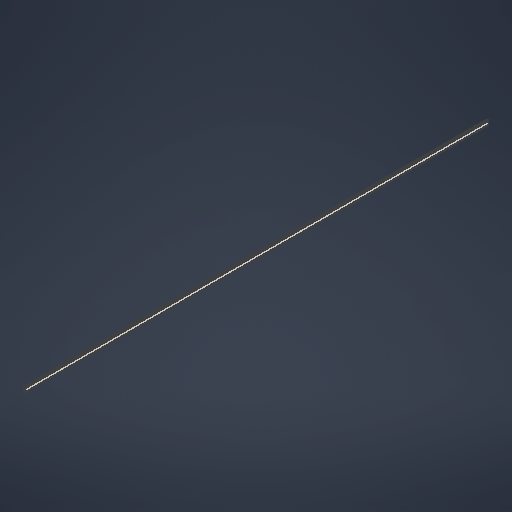
# Autodesk Inventor part: SP40-04A TRAVESAÑO CENTRAL
Saved by Autodesk Inventor 2025 (Build 290162000, 162)
## iProperties
Created: 2026-01-20
Part Number: SP40-04A TRAVESAÑO CENTRAL
Material: Aluminio
Document SubType Name: Modeling
Designer: ROLANDO
Density: 2.7 g/cm^3
Appearance: Satinado
Author: ROLANDO
Autodesk Inventor part; units mm, degrees
ref_plane "YZ Plane" through (0, 0, 0) normal (1, 0, 0) x (0, 1, 0)
ref_plane "XZ Plane" through (0, 0, 0) normal (0, 1, 0) x (-1, 0, 0)
ref_plane "XY Plane" through (0, 0, 0) normal (0, 0, 1) x (1, 0, 0)
sketch "Boceto1" plane through (0, 0, 0) normal (0, 0, 1) x (1, 0, 0)
  line L0 (-4.7609, 13.4664) -> (-4.7609, -16.5336)
  line L1 (-4.7609, -16.5336) -> (0.4391, -16.5336)
  line L2 (0.4391, -16.5336) -> (0.4391, -14.8936)
  line L3 (-0.9609, -15.1336) -> (-3.3609, -15.1336)
  line L4 (-3.3609, -15.1336) -> (-3.3609, -3.0336)
  line L5 (-2.8609, -2.5336) -> (17.5391, -2.5336)
  line L6 (18.0391, -3.0336) -> (18.0391, -7.2336)
  line L7 (18.0391, -7.2336) -> (14.2391, -7.2336)
  line L8 (14.2391, -7.2336) -> (14.2391, -8.8736)
  line L9 (14.9333, -9.8836) -> (15.6391, -9.8836)
  line L10 (15.6391, -9.8836) -> (15.6391, -8.6336)
  line L11 (15.6391, -8.6336) -> (18.0391, -8.6336)
  line L12 (18.0391, -8.6336) -> (18.0391, -15.1336)
  line L13 (18.0391, -15.1336) -> (15.6391, -15.1336)
  line L14 (15.6391, -15.1336) -> (15.6391, -13.8836)
  line L15 (15.6391, -13.8836) -> (14.9333, -13.8836)
  line L16 (14.2391, -14.8936) -> (14.2391, -16.5336)
  line L17 (14.2391, -16.5336) -> (19.4391, -16.5336)
  line L18 (19.4391, -16.5336) -> (19.4391, 13.4664)
  line L19 (-3.3609, 13.4664) -> (-3.3609, -0.6336)
  line L20 (18.0391, -0.6336) -> (18.0391, 13.4664)
  line L21 (7.3391, 11.7517) -> (7.3391, -2.5336) construction
  arc A0 (6.2391, 3.4216) -> (8.4391, 3.4216) centre (7.3391, 1.5164) ccw
  line L22 (-8.4881, 13.4664) -> (24.4446, 13.4664) construction
  line L23 (4.9522, 1.2664) -> (5.1534, 1.2664)
  line L24 (4.9522, 1.7664) -> (5.1534, 1.7664)
  line L25 (-2.8609, -1.1336) -> (3.8304, -1.1336)
  line L26 (10.8478, -1.1336) -> (17.5391, -1.1336)
  line L27 (4.0797, 1.5164) -> (9.7739, 1.5164) construction
  line L28 (9.726, 1.2664) -> (9.5249, 1.2664)
  line L29 (9.726, 1.7664) -> (9.5249, 1.7664)
  line L30 (7.5891, -0.8706) -> (7.5891, -0.6694)
  line L31 (7.0891, -0.8706) -> (7.0891, -0.6694)
  arc A1 (7.0891, -0.8706) -> (7.5891, -0.8706) centre (7.3391, 1.5164) ccw
  arc A2 (9.726, 1.2664) -> (9.726, 1.7664) centre (7.3391, 1.5164) ccw
  arc A3 (4.9522, 1.7664) -> (4.9522, 1.2664) centre (7.3391, 1.5164) ccw
  circle A4 centre (7.3391, 1.5164) radius 2.4 construction
  line L32 (6.2391, 4.9599) -> (6.2391, 3.4216)
  line L33 (8.4391, 4.9599) -> (8.4391, 3.4216)
  arc A5 (10.4214, -0.3724) -> (8.4391, 4.9599) centre (7.3391, 1.5164) ccw
  arc A6 (6.2391, 4.9599) -> (4.2568, -0.3724) centre (7.3391, 1.5164) ccw
  line L34 (-0.9609, -15.1336) -> (-0.9609, -13.8836)
  line L35 (-0.9609, -13.8836) -> (-0.2551, -13.8836)
  line L36 (-0.2551, -13.8836) -> (0.4391, -14.8936)
  line L37 (14.2391, -8.8736) -> (14.9333, -9.8836)
  line L38 (14.2391, -14.8936) -> (14.9333, -13.8836)
  arc A7 (-2.8609, -2.5336) -> (-3.3609, -3.0336) centre (-2.8609, -3.0336) ccw
  arc A8 (-3.3609, -0.6336) -> (-2.8609, -1.1336) centre (-2.8609, -0.6336) ccw
  arc A9 (17.5391, -1.1336) -> (18.0391, -0.6336) centre (17.5391, -0.6336) ccw
  arc A10 (18.0391, -3.0336) -> (17.5391, -2.5336) centre (17.5391, -3.0336) ccw
  arc A11 (3.8304, -1.1336) -> (4.2568, -0.3724) centre (3.8304, -0.6336) ccw
  arc A12 (10.4214, -0.3724) -> (10.8478, -1.1336) centre (10.8478, -0.6336) ccw
  line L39 (-4.7609, 13.4664) -> (-4.7609, 43.4664)
  line L40 (-4.7609, 43.4664) -> (0.4391, 43.4664)
  line L41 (0.4391, 43.4664) -> (0.4391, 41.8264)
  line L42 (-0.9609, 42.0664) -> (-3.3609, 42.0664)
  line L43 (-3.3609, 42.0664) -> (-3.3609, 29.9664)
  line L44 (-2.8609, 29.4664) -> (17.5391, 29.4664)
  line L45 (18.0391, 29.9664) -> (18.0391, 34.1664)
  line L46 (18.0391, 34.1664) -> (14.2391, 34.1664)
  line L47 (14.2391, 34.1664) -> (14.2391, 35.8064)
  line L48 (14.9333, 36.8164) -> (15.6391, 36.8164)
  line L49 (15.6391, 36.8164) -> (15.6391, 35.5664)
  line L50 (15.6391, 35.5664) -> (18.0391, 35.5664)
  line L51 (18.0391, 35.5664) -> (18.0391, 42.0664)
  line L52 (18.0391, 42.0664) -> (15.6391, 42.0664)
  line L53 (15.6391, 42.0664) -> (15.6391, 40.8164)
  line L54 (15.6391, 40.8164) -> (14.9333, 40.8164)
  line L55 (14.2391, 41.8264) -> (14.2391, 43.4664)
  line L56 (14.2391, 43.4664) -> (19.4391, 43.4664)
  line L57 (19.4391, 43.4664) -> (19.4391, 13.4664)
  line L58 (-3.3609, 13.4664) -> (-3.3609, 27.5664)
  line L59 (18.0391, 27.5664) -> (18.0391, 13.4664)
  line L60 (7.3391, 15.181) -> (7.3391, 29.4664) construction
  arc A13 (8.4391, 23.5111) -> (6.2391, 23.5111) centre (7.3391, 25.4164) ccw
  line L61 (4.9522, 25.6664) -> (5.1534, 25.6664)
  line L62 (4.9522, 25.1664) -> (5.1534, 25.1664)
  line L63 (-2.8609, 28.0664) -> (3.8304, 28.0664)
  line L64 (10.8478, 28.0664) -> (17.5391, 28.0664)
  line L65 (4.0797, 25.4164) -> (9.7739, 25.4164) construction
  line L66 (9.726, 25.6664) -> (9.5249, 25.6664)
  line L67 (9.726, 25.1664) -> (9.5249, 25.1664)
  line L68 (7.5891, 27.8033) -> (7.5891, 27.6021)
  line L69 (7.0891, 27.8033) -> (7.0891, 27.6021)
  arc A14 (7.5891, 27.8033) -> (7.0891, 27.8033) centre (7.3391, 25.4164) ccw
  arc A15 (9.726, 25.1664) -> (9.726, 25.6664) centre (7.3391, 25.4164) ccw
  arc A16 (4.9522, 25.6664) -> (4.9522, 25.1664) centre (7.3391, 25.4164) ccw
  circle A17 centre (7.3391, 25.4164) radius 2.4 construction
  line L70 (6.2391, 21.9728) -> (6.2391, 23.5111)
  line L71 (8.4391, 21.9728) -> (8.4391, 23.5111)
  arc A18 (8.4391, 21.9728) -> (10.4214, 27.3051) centre (7.3391, 25.4164) ccw
  arc A19 (4.2568, 27.3051) -> (6.2391, 21.9728) centre (7.3391, 25.4164) ccw
  line L72 (-0.9609, 42.0664) -> (-0.9609, 40.8164)
  line L73 (-0.9609, 40.8164) -> (-0.2551, 40.8164)
  line L74 (-0.2551, 40.8164) -> (0.4391, 41.8264)
  line L75 (14.2391, 35.8064) -> (14.9333, 36.8164)
  line L76 (14.2391, 41.8264) -> (14.9333, 40.8164)
  arc A20 (-3.3609, 29.9664) -> (-2.8609, 29.4664) centre (-2.8609, 29.9664) ccw
  arc A21 (-2.8609, 28.0664) -> (-3.3609, 27.5664) centre (-2.8609, 27.5664) ccw
  arc A22 (18.0391, 27.5664) -> (17.5391, 28.0664) centre (17.5391, 27.5664) ccw
  arc A23 (17.5391, 29.4664) -> (18.0391, 29.9664) centre (17.5391, 29.9664) ccw
  arc A24 (4.2568, 27.3051) -> (3.8304, 28.0664) centre (3.8304, 27.5664) ccw
  arc A25 (10.8478, 28.0664) -> (10.4214, 27.3051) centre (10.8478, 27.5664) ccw
  point P0 (4.8803, -1.1336)
  point P1 (9.7979, -1.1336)
  point P2 (7.3391, -2.5336)
  point P3 (18.0391, -11.8836)
  point P4 (4.8803, 28.0664)
  point P5 (9.7979, 28.0664)
  point P6 (7.3391, 29.4664)
  point P7 (18.0391, 38.8164)
  dimension "d0" = 1.4
  dimension "d1" = 1.4
  dimension "d2" = 1.4
  dimension "d3" = 1.4
  dimension "d4" = 1.4
  dimension "d5" = 1.4
  dimension "d6" = 1.4
  dimension "d7" = 1.4
  dimension "d8" = 1.4
  dimension "d9" = 1.4
  dimension "d12" = 4.4
  dimension "d19" = 0.5
  dimension "d22" = 4.05
  dimension "d24" = 0.25
  dimension "d25" = 0.25
  dimension "d26" = 0.5
  dimension "d30" = 0.5
  dimension "d32" = 4.8
  dimension "d35" = 1.1
  dimension "d36" = 2.2
  dimension "d37" = 1.415
  dimension "d38" = 1.415
  dimension "d39" = 0.2
  dimension "d40" = 0.2
  dimension "d42" = 30
  dimension "d43" = 14
  dimension "d44" = 4
  dimension "d45" = 9.3
  dimension "d46" = 6.5
  dimension "d47" = 24.2
  dimension "d48" = 5.2
  dimension "d49" = 1.4
  dimension "d50" = 5.2
  dimension "d51" = 13.8
  dimension "d52" = 21.4
  dimension "d53" = 0.2
  dimension "d55" = 0.2
  dimension "d56" = 0.25
  dimension "d57" = 0.2
  dimension "d58" = 1.4
  dimension "d62" = 1.4
  dimension "d63" = 2.65
  dimension "d64" = 1.64
  dimension "d65" = 34.5
  dimension "d66" = 2
  dimension "d67" = 2
  dimension "d68" = 2.4
  dimension "d69" = 3.01
  dimension "d70" = 6.02
  dimension "d71" = 34.5
  dimension "d72" = 111
  dimension "d74" = 0.7058
  dimension "d75" = 0.7058
  dimension "d82" = 9.6652
  dimension "d83" = 25.6354
  dimension "d84" = 15.3594
  dimension "d86" = 0.5
  dimension "d87" = 0.5
  dimension "d88" = 60
  dimension "d89" = 30.6
  constraints: 154 end point, 67 symmetric about line, 64 point on circle, 26 centre point, 18 perpendicular, 14 point on line, 12 tangent, 7 collinear, 7 vertical, 6 coincident, 4 equal radius, 4 midpoint, 4 parallel, 3 horizontal, 13 other
  measures "d0" distance between parallel lines of L19 L0
  measures "d1" distance between parallel lines of L0 L4
  measures "d2" distance between parallel lines of L1 L3
  measures "d3" distance between parallel lines of L18 L20
  measures "d4" distance between parallel lines of L18 L6
  measures "d5" distance between parallel lines of L18 L12
  measures "d6" distance between parallel lines of L17 L13
  measures "d7" distance between parallel lines of L7 L11
  measures "d8" distance between parallel lines of L8 L10
  measures "d9" distance between parallel lines of L16 L14
  measures "d12" diameter of A0
  measures "d19" distance between parallel lines of L23 L24
  measures "d22" distance from line of A5.centre L5
  measures "d24" distance between parallel lines of L24 L27
  measures "d25" distance between parallel lines of L27 L29
  measures "d26" distance between parallel lines of L28 L29
  measures "d30" distance between parallel lines of L31 L30
  measures "d32" diameter of A4
  measures "d35" distance between parallel lines of L21 L32
  measures "d36" distance between parallel lines of L33 L32
  measures "d37" radial gap between concentric circles of A0 A5
  measures "d38" radial gap between concentric circles of A6 A0
  measures "d39" radial gap between concentric circles of A4 A0
  measures "d40" radial gap between concentric circles of A4 A0
  measures "d42" distance between parallel lines of L17 L22
  measures "d43" distance between parallel lines of L17 L5
  measures "d44" distance between parallel lines of L15 L9
  measures "d45" distance between parallel lines of L17 L7
  measures "d46" distance between parallel lines of L13 L11
  measures "d47" distance between parallel lines of L18 L0
  measures "d48" distance between parallel lines of L0 L2
  measures "d49" distance between parallel lines of L2 L34
  measures "d50" distance between parallel lines of L18 L16
  measures "d51" distance between parallel lines of L2 L16
  measures "d52" distance between parallel lines of L12 L4
  measures "d53" radial gap between concentric circles of A0 A3
  measures "d55" radial gap between concentric circles of A1 A0
  measures "d56" distance between parallel lines of L30 L21
  measures "d57" radial gap between concentric circles of A2 A0
  measures "d58" distance between parallel lines of L5 L26
  measures "d62" distance between parallel lines of L5 L25
  measures "d63" distance between parallel lines of L35 L1
  measures "d64" distance of L1.end L2.end
  measures "d65" angle of L2 L36
  measures "d66" distance from line of point (18.039, -11.884) L9
  measures "d67" distance from line of point (18.039, -11.884) L15
  measures "d68" distance between parallel lines of L12 L10
  measures "d69" vertical distance of point (18.039, -11.884) L8.end
  measures "d70" distance of L8.end L16.start
  measures "d71" angle of L10 L37
  measures "d72" angle of L38 L37
  measures "d74" distance of L9.start L9.end
  measures "d75" distance of L14.end L15.end
  measures "d82" distance from line of L27.end L18
  measures "d83" distance from line of L21.start L15
  measures "d84" distance from line of L27.start L18
  measures "d86" radius of A7
  measures "d87" radius of A8
  measures "d88" distance between parallel lines of L17 L56
  measures "d89" distance between parallel lines of L26 L44
extrude "Extrusión1" add sketch "Boceto1" against normal blind 5800
